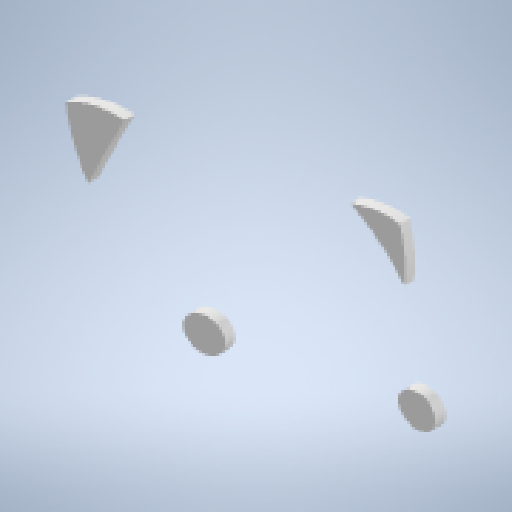
# Autodesk Inventor part: CheeksEarsGoma
Saved by Autodesk Inventor 2023 (Build 270158000, 158)
## iProperties
Created: 2022-11-10
Part Number: CheeksEarsGoma
Material: Generic
Document SubType Name: Modeling
Designer: reide
Density: 1 g/cm^3
Appearance: Default
Author: reide
Autodesk Inventor part; units mm, degrees
ref_plane "YZ Plane" through (0, 0, 0) normal (1, 0, 0) x (0, 1, 0)
ref_plane "XZ Plane" through (0, 0, 0) normal (0, 1, 0) x (-1, 0, 0)
ref_plane "XY Plane" through (0, 0, 0) normal (0, 0, 1) x (1, 0, 0)
sketch "Sketch1" plane through (0, 0, 0) normal (0, 0, 1) x (1, 0, 0)
  arc A0 (39.4707, -22.8264) -> (44.1913, -18.1315) centre (29.9144, -8.4969) ccw projected
  arc A1 (44.1913, -18.1315) -> (43.1493, -16.8575) centre (-1.7028, -54.6052) ccw projected
  line L0 (39.4808, -21.8264) -> (5.243, -21.8264) projected
  arc A2 (5.243, -21.8264) -> (4.9829, -20.5171) centre (3.1145, -21.5688) ccw projected
  arc A3 (4.9829, -20.5171) -> (7.1052, -17.9527) centre (4.0499, -17.5844) ccw projected
  arc A4 (7.1052, -17.9527) -> (35.9599, -11.4954) centre (11.3687, 30.6937) ccw projected
  arc A5 (43.1493, -16.8575) -> (46.7596, -12.3801) centre (22.9538, 3.1213) ccw projected
  arc A6 (37.9906, -11.4185) -> (42.4917, -16.1906) centre (50.7047, -3.9352) ccw projected
  arc A7 (37.9906, -11.4185) -> (40.4851, -9.7622) centre (30.9595, 1.8767) ccw projected
  arc A8 (44.5875, -12.9722) -> (40.4851, -9.7622) centre (42.1356, -11.8793) ccw projected
  arc A9 (46.7596, -12.3801) -> (45.5083, -8.9416) centre (44.5544, -11.2357) ccw projected
  arc A10 (44.6424, -5.9416) -> (45.5083, -8.9416) centre (46.2763, -7.0949) ccw projected
  arc A11 (44.6424, -5.9416) -> (44.0119, 11.0781) centre (33.1722, 2.155) ccw projected
  arc A12 (44.0119, 11.0781) -> (39.7722, 25.0886) centre (15.7574, 10.1749) ccw projected
  arc A13 (39.7722, 25.0886) -> (38.7065, 38.8808) centre (8.3038, 29.5944) ccw projected
  arc A14 (38.7065, 38.8808) -> (25.3942, 36.764) centre (35.104, 18.6189) ccw projected
  arc A15 (25.3942, 36.764) -> (-13.8323, 30.1524) centre (11.651, -1.3685) ccw projected
  arc A16 (-13.8323, 30.1524) -> (-28.7918, 26.8989) centre (-15.8151, 3.2509) ccw projected
  arc A17 (-28.7918, 26.8989) -> (-24.9989, 11.3281) centre (26.001, 31.9986) ccw projected
  arc A18 (-24.9989, 11.3281) -> (-21.9925, -9.8739) centre (11.0237, 5.6218) ccw projected
  arc A19 (-21.9925, -9.8739) -> (-9.9108, -18.9877) centre (-5.532, -0.6178) ccw projected
  arc A20 (-9.9108, -18.9877) -> (-9.9382, -22.8264) centre (-3.5885, -20.9522) ccw projected
  line L1 (-36.0285, -22.8264) -> (-9.9382, -22.8264) projected
  arc A21 (-36.0285, -22.8264) -> (-40.0285, -26.8264) centre (-36.0285, -26.8264) ccw projected
  line L2 (-40.0285, -131.8264) -> (-40.0285, -26.8264) projected
  arc A22 (-40.0285, -131.8264) -> (-36.0285, -135.8264) centre (-36.0285, -131.8264) ccw projected
  line L3 (101.1727, -135.8264) -> (-36.0285, -135.8264) projected
  line L4 (101.1727, -127.8248) -> (101.1727, -135.8264) projected
  line L5 (-30.6035, -127.8248) -> (101.1727, -127.8248) projected
  arc A23 (-32.6035, -125.8248) -> (-30.6035, -127.8248) centre (-30.6035, -125.8248) ccw projected
  line L6 (-32.6035, -32.8264) -> (-32.6035, -125.8248) projected
  arc A24 (-30.6035, -30.8264) -> (-32.6035, -32.8264) centre (-30.6035, -32.8264) ccw projected
  line L7 (101.1727, -30.8264) -> (-30.6035, -30.8264) projected
  line L8 (101.1727, -22.8264) -> (101.1727, -30.8264) projected
  line L9 (39.4707, -22.8264) -> (101.1727, -22.8264) projected
  arc A25 (18.7696, 4.6569) -> (17.7037, 4.7458) centre (18.2404, 4.7458) ccw projected
  arc A26 (18.7696, 4.6569) -> (18.909, 4.2605) centre (19.3843, 4.6504) ccw projected
  arc A27 (18.909, 4.2605) -> (20.5255, 4.6689) centre (19.5973, 4.9394) ccw projected
  arc A28 (22.3746, 4.7458) -> (20.5255, 4.6689) centre (21.468, 4.2743) ccw projected
  arc A29 (22.3746, 4.7458) -> (23.8239, 5.6218) centre (22.9311, 5.4619) ccw projected
  arc A30 (24.9097, 5.9816) -> (23.8239, 5.6218) centre (24.3471, 5.8612) ccw projected
  arc A31 (21.4025, 4.0439) -> (24.9097, 5.9816) centre (22.9819, 5.328) ccw projected
  arc A32 (17.7037, 4.7458) -> (21.4025, 4.0439) centre (19.5995, 4.6393) ccw projected
  arc A33 (38.9434, 27.1055) -> (27.9206, 36.1462) centre (15.299, 9.5172) ccw projected
  arc A34 (38.0735, 37.6007) -> (27.9206, 36.1462) centre (35.6221, 18.5499) ccw projected
  arc A35 (38.9434, 27.1055) -> (38.0735, 37.6007) centre (11.0038, 30.0735) ccw projected
  line L10 (0.8426, -21.8264) -> (-9.2354, -21.8264) projected
  arc A36 (-0.9, -12.3459) -> (-7.4967, -15.4462) centre (1.4985, -26.0176) ccw projected
  arc A37 (3.3173, -20.9522) -> (-0.9, -12.3459) centre (-13.3261, -23.7716) ccw projected
  arc A38 (3.3173, -20.9522) -> (0.8426, -21.8264) centre (10.6872, -45.7558) ccw projected
  circle A39 centre (33.1722, 9.6232) radius 3.1762 projected
  circle A40 centre (8.3038, 4.7458) radius 3.3209 projected
  arc A41 (-14.9985, 28.4852) -> (-22.4029, 13.6552) centre (214.1169, -95.1731) ccw projected
  arc A42 (-26.9068, 25.7639) -> (-22.4029, 13.6552) centre (-2.3081, 28.0214) ccw projected
  arc A43 (-14.9985, 28.4852) -> (-26.9068, 25.7639) centre (-16.4507, 7.4242) ccw projected
  arc A44 (4.5384, -18.7873) -> (1.4985, -12.8876) centre (3.1669, -15.761) ccw projected
  arc A45 (4.5384, -18.7873) -> (1.4985, -12.8876) centre (-6.3378, -20.6585) ccw projected
  ellipse E0 centre (41.2193, 7.7824) end of major axis (44.9987, 7.7824) minor radius 3.3363 projected
  ellipse E1 centre (0, 0) end of major axis (4.2825, 0.9624) minor radius 3.3846 projected
  ellipse E2 centre (41.2193, 7.7824) end of major axis (37.6335, 7.6225) minor radius 3.1683
  ellipse E3 centre (0, 0) end of major axis (-3.948, -1.3) minor radius 3.2131
  arc A46 (38.7773, 27.466) -> (28.3057, 36.0547) centre (16.3151, 10.7572) ccw
  arc A47 (38.7773, 27.466) -> (37.951, 37.4364) centre (12.2347, 30.2856) ccw
  arc A48 (37.951, 37.4364) -> (28.3057, 36.0547) centre (35.6221, 19.3382) ccw
  arc A49 (-15.355, 28.1902) -> (-26.6679, 25.605) centre (-16.7346, 8.1823) ccw
  arc A50 (-26.6679, 25.605) -> (-22.3892, 14.1017) centre (-3.2991, 27.7497) ccw
  arc A51 (-15.355, 28.1902) -> (-22.3892, 14.1017) centre (202.3047, -89.2851) ccw
  arc A52 (42.4917, -16.1906) -> (44.5875, -12.9722) centre (34.8579, -8.9279) ccw projected
  arc A53 (35.9599, -11.4954) -> (42.2286, -18.7873) centre (49.0814, -6.5556) ccw projected
  arc A54 (39.4808, -21.8264) -> (42.2286, -18.7873) centre (23.3805, -4.507) ccw projected
  arc A55 (-7.4967, -15.4462) -> (-9.2354, -21.8264) centre (-3.1993, -20.0443) ccw projected
  point P0 (35.6221, 34.316)
  point P1 (-22.1282, 22.5866)
  constraints: 12 point on circle, 6 centre point, 2 coincident, 4 other
extrude "Extrusion1" add sketch "Sketch1" along normal blind 2 contours E2 | E3 | A46 A48 A47 | A51 A50 A49
body "Solid1"
